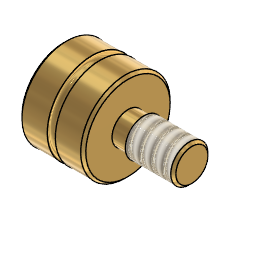
Fire Piston (Autodesk Fusion 360 archive; units mm, degrees)
design "Piston End"
part number: 2026-06-23-20-43-56-503
Autodesk Fusion 360 part; units mm, degrees
sketch "Sketch1" plane through (0, 0, 0) normal (0, 1, 0) x (1, 0, 0)
  line L0 (-0.5, 0) -> (0.5, 0)
  line L1 (0.5, 0) -> (0.5, -0.1565)
  line L2 (0.5, -0.1565) -> (0.125, -0.1565)
  line L3 (0.125, -0.1565) -> (0.125, -0.125)
  line L4 (0.125, -0.125) -> (0, -0.125)
  line L5 (0, -0.125) -> (0, -0.35)
  line L6 (0, -0.35) -> (-0.5, -0.35)
  line L7 (-0.5, -0.35) -> (-0.5, 0)
  circle A0 centre (-0.25, -0.35) radius 0.0315
  dimension "d1" = 0.063
  dimension "d2" = 0.5
  dimension "d3" = 0.5
  dimension "d4" = 0.125
  dimension "d5" = 0.313
  dimension "d6" = 0.25
  dimension "d7" = 0.7
  constraint horizontal L0
  constraint perpendicular L0 L1
  constraint perpendicular L1 L2
  constraint perpendicular L2 L3
  constraint perpendicular L3 L4
  constraint perpendicular L4 L5
  constraint perpendicular L5 L6
  constraint vertical L7
  constraint coincident origin L5
  constraint coincident origin L0
  constraint midpoint L6 A0.centre
  measures "d1" diameter of A0
  measures "d2" distance of L5.end L6.end
  measures "d3" distance of L1 L5
  measures "d4" distance of L3.end L4.end
revolve "Revolve1" add sketch "Sketch1" angle 360 about axis through (-0.5, 0, 0) along (1, 0, 0) contours L0 L1 L2 L3 L4 L5 L6 L7 A0
chamfer "Chamfer1" distance 0.02 angle 45 3 edges at (-0.5, -0.1266, -0.3263) (0, -0.1266, -0.3263) (0.5, -0.0566, -0.1459)
thread "Thread1" "ISO Metric profile 0.3 M0.3x0.09 M0.3x0.09 6g" major diameter 0.2915 minor diameter 0.181 pitch 0.09 angle 60 resizes the face on face at (0.2433, 0.0156, 0.1557)

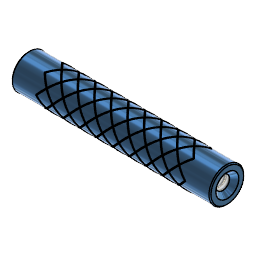
design "Piston Body"
part number: 2026-06-23-18-50-12-006
Autodesk Fusion 360 part; units mm, degrees
derive "DerivedContext1" from "Fire Piston v1"
sketch "Sketch1" plane through (0, 0, 0) normal (0, 1, 0) x (1, 0, 0)
  line L0 (0, -0.35) -> (4, -0.35)
  line L1 (4, -0.35) -> (4, -0.175)
  line L2 (4, -0.175) -> (3.5, -0.175)
  line L3 (3.5, -0.175) -> (3.5, -0.1953)
  line L4 (3.5, -0.1953) -> (0, -0.1953)
  line L5 (0, -0.1953) -> (0, -0.35)
  line L6 (0, 0) -> (4, 0)
  dimension "d1" = 4
  dimension "d2" = 0.5
  dimension "d3" = 0.35
  dimension "d4" = 0.7
  dimension "d5" = 0.3906
  constraint horizontal L0
  constraint perpendicular L0 L1
  constraint perpendicular L1 L2
  constraint perpendicular L2 L3
  constraint perpendicular L1 L4
  constraint perpendicular L0 L5
  constraint coincident L6.start origin
  constraint horizontal L6
  constraint coincident L6.start L5
  constraint coincident L1 L6.end
  measures "d1" distance of L0.start L0.end
  measures "d2" distance of L1.end L2.end
revolve "Revolve1" add sketch "Sketch1" angle 360 about axis through (0, 0, 0) along (1, 0, 0)
thread "Thread1" "ISO Metric profile 0.35 M0.35x0.09 M0.35x0.09 6H" major diameter 0.368 minor diameter 0.2765 pitch 0.09 angle 60 resizes the face on face at (3.8333, 0.0087, 0.1748)
chamfer "Chamfer1" distance 0.0938 angle 45 1 edges at (4, -0.05, -0.1289)
chamfer "Chamfer1" distance 0.02 angle 45 1 edges at (4, -0.1266, -0.3263) 1 faces at (0, 0.0174, 0.2971)
ref_plane "WorkPlane1" through (0.5, 0, 0) normal (-1, 0, 0) x (0, 0, 1)
coil "CoilPrimitive1" cut diameter 0.7 section triangle in size 0.02 inside turns 1.5 pitch 2 right hand placed x (0, -1, 0) y (0, 0, -1) z (1, 0, 0) at (0.5, 0, 0)
mirror "Mirror1" about plane through (0, 0, 0) normal (0, 1, 0) of "CoilPrimitive1"
pattern_circular "C-Pattern1" count 6 over 360 about axis through (3.5, 0, 0) along (-1, 0, 0) of "CoilPrimitive1", "Mirror1"
equation "d5 = ( 25 / 64 ) * 1 mm"
equation "d9 = ( 3 / 32 ) * 1 mm"

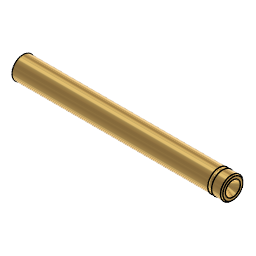
design "Piston"
part number: 2026-06-23-20-51-12-808
Autodesk Fusion 360 part; units mm, degrees
sketch "Sketch1" plane through (0, 0, 0) normal (0, 1, 0) x (1, 0, 0)
  line L0 (0, 0) -> (3.5, 0)
  line L1 (3.5, 0) -> (3.5, -0.1875)
  line L2 (3.5, -0.1875) -> (0, -0.1875)
  line L3 (0, -0.1875) -> (0, 0)
  circle A0 centre (3.3, -0.1875) radius 0.0312
  dimension "d1" = 0.0625
  dimension "d2" = 0.2
  dimension "d3" = 0.375
  dimension "d4" = 3.5
  constraint horizontal L0
  constraint vertical L1
  constraint horizontal L2
  constraint vertical L3
  constraint coincident L0.start L3.end
  constraint coincident L2 A0.centre
  measures "d1" diameter of A0
  measures "d2" distance of L1 A0.centre
  measures "d4" distance of L1.end L2.end
revolve "Revolve1" add sketch "Sketch1" angle 360 about axis through (0, 0, 0) along (1, 0, 0) contours L0 L1 L2 L3 A0
hole "Hole1" at (3.5, 0, 0) direction (-1, 0, 0) diameter 0.0556 depth 0.1875 tip angle 118 countersink diameter 0.25 countersink angle 82
chamfer "Chamfer1" distance 0.02 angle 45 1 edges at (3.5, -0.0678, -0.1748)
hole "Hole2" at (0, -0.0041, -0.0014) direction (1, 0, 0) diameter 0.19 depth 0.5 tip angle 118
thread "Thread1" "ISO Metric profile 0.25 M0.25x0.075 M0.25x0.075 6H" thread offset 0 thread depth 7.4
equation "d1 = ( 1 / 16 ) * 1 mm"
equation "d3 = ( 3 / 8 ) * 1 mm"
equation "d6 = ( 3 / 16 ) * 1 mm"
equation "d7 = ( 1 / 18 ) * 1 mm"

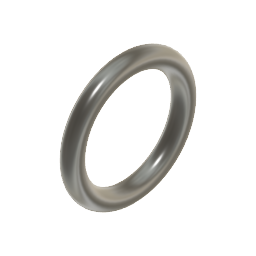
design "ring"
part number: 2026-06-23-19-53-18-470
Autodesk Fusion 360 part; units mm, degrees
other "DerivedContext1"
sketch "Sketch4" plane through (0, 0, 0) normal (0, 1, 0) x (1, 0, 0)
  circle A0 centre (4.961, 0.2343) radius 0.0385
revolve "Revolve1" add sketch "Sketch4" angle 360 about axis through (1.75, 0, 0) along (1, 0, 0)
